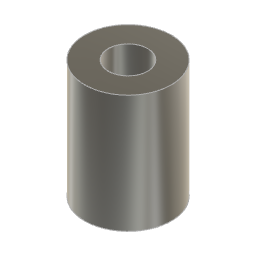
_Tape Roller.82510a13-c087-4876-a560-cccf8a565558 (Autodesk Fusion 360 design; units mm, degrees)
Autodesk Fusion 360 part; units mm, degrees
sketch "Sketch1" plane through (0, 0, 0) normal (0, 0, 1) x (1, 0, 0)
  circle A0 centre (0, 0) radius 6.985
  circle A1 centre (0, 0) radius 3.175
  dimension "d1" = 13.97
  dimension "d2" = 6.35
  constraint coincident A0.centre A1.centre
  measures "d1" diameter of A0
  measures "d2" diameter of A1
extrude "Extrude1" add sketch "Sketch1" along normal blind 19.05
